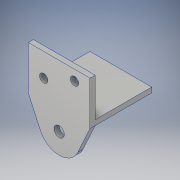
# Autodesk Inventor part: CLB_087_ClimberMountBracketGusset
Saved by Autodesk Inventor 2018 (Build 220112000, 112)
## iProperties
Created: 2020-02-22
Part Number: CLB_087_ClimberMountBracketGusset
Material: Aluminum 6061
Document SubType Name: Modeling
Designer: 22perngrac
Density: 2.7 g/cm^3
Appearance: Aluminum - Flat
Mass: 21.4358 g
Surface Area: 58.1692 cm^2
Volume: 7.93919 cm^3
Author: 22perngrac
Autodesk Inventor part; units mm, degrees
ref_plane "YZ Plane" through (0, 0, 0) normal (1, 0, 0) x (0, 1, 0)
ref_plane "XZ Plane" through (0, 0, 0) normal (0, 1, 0) x (-1, 0, 0)
ref_plane "XY Plane" through (0, 0, 0) normal (0, 0, 1) x (1, 0, 0)
sketch "Sketch1" plane through (0, 0, 0) normal (0, 0, 1) x (1, 0, 0)
  line L0 (0, 0) -> (38.1, 0)
  line L1 (38.1, 0) -> (38.1, -26.9875)
  line L2 (0, 0) -> (0, -26.9875)
  line L3 (0, -26.9875) -> (7.5012, -43.3836)
  line L4 (38.1, -26.9875) -> (30.5988, -43.3836)
  arc A0 (7.5012, -43.3836) -> (30.5988, -43.3836) centre (19.05, -38.1) ccw
  line L5 (38.1, -25.4) -> (0, -25.4) construction
  line L6 (38.1, -26.9875) -> (0, -26.9875) construction
  line L7 (38.1, -23.8125) -> (0, -23.8125) construction
  dimension "d1" = 38.1
  dimension "d2" = 12.7
  dimension "d36" = 38.1
  dimension "d37" = 25.4
  dimension "d38" = 1.5875
  dimension "d39" = 1.5875
  constraints: 16 end point, 7 point on line, 4 perpendicular, 2 equal length, 2 point on circle, 2 tangent, 1 centre point, 1 horizontal, 1 vertical
  measures "d1" distance of L0.start L0.end
  measures "d2" radius of A0
  measures "d36" distance from line of L0 A0.centre
  measures "d37" distance between parallel lines of L0 L5
  measures "d38" distance between parallel lines of L5 L6
  measures "d39" distance between parallel lines of L5 L7
extrude "Extrusion1" add sketch "Sketch1" along normal blind 3.175
sketch "Sketch2" plane through (0, 0, 0) normal (0, 0, -1) x (-1, 0, 0)
  line L0 (-38.1, 0) -> (-38.1, -26.9875) projected
  line L1 (0, -26.9875) -> (0, 0) projected
  line L2 (-38.1, -26.9875) -> (0, -26.9875)
  line L3 (0, -26.9875) -> (0, -23.8125)
  line L4 (0, -23.8125) -> (-38.1, -23.8125)
  line L5 (-38.1, -23.8125) -> (-38.1, -26.9875)
  arc A0 (-7.5012, -43.3836) -> (-30.5988, -43.3836) centre (-19.05, -38.1) ccw projected
  dimension "d13" = 3.175
  constraints: 8 end point, 2 parallel, 1 horizontal, 1 perpendicular, 1 point on line
  measures "d13" distance between parallel lines of L2 L4
extrude "Extrusion2" add sketch "Sketch2" along normal blind 34.925
sketch "Sketch3" plane through (0, 0, 3.175) normal (0, 0, 1) x (1, 0, 0)
  line L0 (7.5012, -43.3836) -> (0, -26.9875) projected
  arc A0 (30.5988, -43.3836) -> (7.5012, -43.3836) centre (19.05, -38.1) ccw projected
  line L1 (0, -26.9875) -> (0, 0) projected
  line L2 (0, 0) -> (38.1, 0) projected
  line L3 (38.1, 0) -> (38.1, -26.9875) projected
  line L4 (38.1, -23.8125) -> (0, -23.8125) projected
  line L5 (38.1, -23.8125) -> (0, -23.8125) projected
  point P0 (9.525, -14.2875)
  point P1 (28.575, -6.35)
  dimension "d18" = 9.525
  dimension "d20" = 6.35
  dimension "d21" = 9.525
  dimension "d40" = 9.525
  measures "d18" distance from line of L1 point (9.525, -14.288)
  measures "d20" distance from line of point (28.575, -6.35) L2
  measures "d21" distance from line of L3 point (28.575, -6.35)
  measures "d40" distance from line of L4 point (9.525, -14.288)
hole "Hole1" at (9.525, -14.2875, 3.175) at (28.575, -6.35, 3.175) direction (0, 0, -1) diameter 5.1054 end through all clearance for "Flat Head Machine Screw (82)" size "#10" standard "Ansi Unified Screw Threads"
sketch "Sketch4" plane through (0, 0, 3.175) normal (0, 0, 1) x (1, 0, 0)
  arc A0 (30.5988, -43.3836) -> (7.5012, -43.3836) centre (19.05, -38.1) ccw projected
  point P0 (0, 0)
  constraints: 1 coincident
hole "Hole2" at (19.05, -38.1, 3.175) direction (0, 0, -1) diameter 6.35 end through all
body "Solid1"
